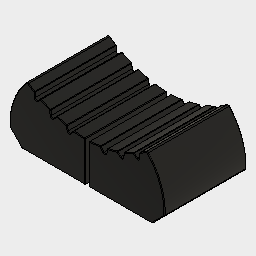
ALPS Fader Knob (Autodesk Fusion 360 design; units mm, degrees)
Autodesk Fusion 360 part; units mm, degrees
sketch "Skizze1" plane through (0, 0, 0) normal (0, 1, 0) x (1, 0, 0)
  line L0 (0, 0) -> (10.3, 0)
  line L1 (10.3, 0) -> (12.3, -2)
  line L2 (0, -11.0044) -> (0, 4.9956) construction
  arc A0 (9.5, -9.5) -> (12.3, -2) centre (1.806, -2.3549) ccw
  arc A1 (9.5, -9.5) -> (0, -6.3) centre (-0.6023, -23.7896) ccw
  line L3 (-0.9062, -6.3) -> (0.9938, -6.3) construction
  arc A2 (-12.3, -2) -> (-9.5, -9.5) centre (-1.806, -2.3549) ccw
  arc A3 (0, -6.3) -> (-9.5, -9.5) centre (0.6023, -23.7896) ccw
  line L4 (0, 0) -> (-10.3, 0)
  line L5 (-10.3, 0) -> (-12.3, -2)
  dimension "d1" = 135
  dimension "d2" = 6.3
  dimension "d3" = 2
  dimension "d4" = 10.3
  dimension "d5" = 10.5
  dimension "d6" = 17.5
  dimension "d7" = 9.5
  dimension "d8" = 9.5
  measures "d1" angle of L0 L1
  measures "d2" distance of L0.start L3
  measures "d3" distance of L0 L1.end
  measures "d4" distance of L0.start L0.end
  measures "d5" radius of A0
  measures "d6" radius of A1
  measures "d7" distance of L2 A0.start
  measures "d8" distance of L0 A0.start
extrude "Extrusion1" add sketch "Skizze1" along normal mid plane 13
sketch "Skizze2" plane through (0, -6.5, 0) normal (0, -1, 0) x (1, 0, 0)
  line L0 (-10.3, 0) -> (10.3, 0)
  line L1 (10.3, 0) -> (12.3, 2)
  arc A0 (12.3, 2) -> (9.5, 9.5) centre (1.806, 2.3549) ccw
  arc A1 (0, 6.3) -> (9.5, 9.5) centre (-0.6023, 23.7896) ccw
  arc A2 (-9.5, 9.5) -> (0, 6.3) centre (0.6023, 23.7896) ccw
  arc A3 (-9.5, 9.5) -> (-12.3, 2) centre (-1.806, 2.3549) ccw
  line L2 (-12.3, 2) -> (-10.3, 0)
  arc A4 (-9.5, 9.5) -> (0, 6.3) centre (0.6023, 23.7896) ccw
  arc A5 (0, 6.3) -> (9.5, 9.5) centre (-0.6023, 23.7896) ccw
  line L3 (10.3, 0) -> (-10.3, 0)
  line L4 (-10.3, 0) -> (-12.3, 2)
  arc A6 (-9.5, 9.5) -> (-12.3, 2) centre (-1.806, 2.3549) ccw
  arc A7 (-9.5, 9.5) -> (0, 6.3) centre (0.6023, 23.7896) ccw
  arc A8 (0, 6.3) -> (9.5, 9.5) centre (-0.6023, 23.7896) ccw
  arc A9 (12.3, 2) -> (9.5, 9.5) centre (1.806, 2.3549) ccw
  line L5 (12.3, 2) -> (10.3, 0)
  line L6 (-8.3055, 8.7264) -> (-8.2923, 7.9551)
  line L7 (-7.8783, 7.7707) -> (-7.3709, 8.2115)
  arc A10 (-8.2923, 7.9551) -> (-7.8783, 7.7707) centre (-8.0423, 7.9594) ccw
  line L8 (-5.8203, 7.5108) -> (-5.7421, 6.772)
  arc A11 (-5.7421, 6.772) -> (-5.3135, 6.6248) centre (-5.4935, 6.7983) ccw
  line L9 (-5.3135, 6.6248) -> (-4.8095, 7.1475)
  line L10 (-2.6202, 5.8954) -> (-2.1282, 6.504)
  arc A12 (-3.06, 6.0046) -> (-2.6202, 5.8954) centre (-2.8147, 6.0525) ccw
  line L11 (-3.1972, 6.7071) -> (-3.06, 6.0046)
  line L12 (-0.35, 6.3156) -> (-0.35, 5.5)
  line L13 (-0.35, 5.5) -> (0.35, 5.5)
  line L14 (0.35, 5.5) -> (0.35, 6.3156)
  line L15 (1.75, 0) -> (22.5, 0)
  line L16 (0, 1.75) -> (0, 22.5)
  line L17 (7.8783, 7.7707) -> (7.3709, 8.2115)
  arc A13 (7.8783, 7.7707) -> (8.2923, 7.9551) centre (8.0423, 7.9594) ccw
  line L18 (8.3055, 8.7264) -> (8.2923, 7.9551)
  line L19 (5.3135, 6.6248) -> (4.8095, 7.1475)
  arc A14 (5.3135, 6.6248) -> (5.7421, 6.772) centre (5.4935, 6.7983) ccw
  line L20 (5.8203, 7.5108) -> (5.7421, 6.772)
  line L21 (2.6202, 5.8954) -> (2.1282, 6.504)
  arc A15 (2.6202, 5.8954) -> (3.06, 6.0046) centre (2.8147, 6.0525) ccw
  line L22 (3.1972, 6.7071) -> (3.06, 6.0046)
  dimension "d12" = 50
  dimension "d13" = 0.25
  dimension "d14" = 50
  dimension "d15" = 0.25
  dimension "d16" = 50
  dimension "d17" = 0.25
  dimension "d18" = 0.8
  dimension "d29" = 0.7
  measures "d12" angle of L6 L7
  measures "d13" radius of A10
  measures "d14" angle of L8 L9
  measures "d15" radius of A11
  measures "d16" angle of L10 L11
  measures "d17" radius of A12
  measures "d18" distance of A1.start L13
  measures "d29" distance of L12 L14
extrude "Extrusion2" cut sketch "Skizze2" against normal blind 13 contours A2 A4 A7 L6 L7 A10 | A1 A5 A8 L17 A13 L18 | A2 A4 A7 L8 A11 L9 | A1 A5 A8 L19 A14 L20 | A2 A4 A7 L10 A12 L11 | A1 A5 A8 L21 A15 L22 | A2 A4 A7 L12 L13 L16 | A1 A5 A8 L13 L14 L16
fillet "Abrundung1" radius 0.1 14 edges at (-8.3055, 0, 8.7264) (-7.3709, 0, 8.2115) (-5.8203, 0, 7.5108) (-4.8095, 0, 7.1475) (-3.1972, 0, 6.7071) (-2.1282, 0, 6.504) (-0.35, 0, 6.3156) (0.35, 0, 6.3156) (2.1282, 0, 6.504) (3.1972, 0, 6.7071) (4.8095, 0, 7.1475) (5.8203, 0, 7.5108) (7.3709, 0, 8.2115) (8.3055, 0, 8.7264)
fillet "Abrundung2" radius 0.25 6 edges at (-9.5, 0, 9.5) (9.5, 0, 9.5) (12.3, 0, 2) (10.3, 0, 0) (-12.3, 0, 2) (-10.3, 0, 0)
sketch "Skizze4" plane through (0, 0, 0) normal (0, 0, 1) x (1, 0, 0)
  line L0 (1.75, 0) -> (22.5, 0)
  line L1 (-0.35, -6.5) -> (0.35, -6.5)
  line L2 (0.35, -6.5) -> (0.35, -5.8)
  line L3 (0.35, -5.8) -> (-0.35, -5.8)
  line L4 (-0.35, -5.8) -> (-0.35, -6.5)
  line L5 (0.35, -6.5) -> (-0.35, -6.5)
  line L6 (-10.1964, -6.5) -> (10.1964, -6.5)
  line L7 (0, 1.75) -> (0, 22.5)
  line L8 (0.35, 6.5) -> (0.35, 5.8)
  line L9 (-0.35, 5.8) -> (-0.35, 6.5)
  line L10 (-0.35, 6.5) -> (0.35, 6.5)
  line L11 (0.35, 6.5) -> (-0.35, 6.5)
  line L12 (-10.1964, 6.5) -> (10.1964, 6.5)
  line L13 (0.35, 5.8) -> (-0.35, 5.8)
  dimension "d25" = 0.7
  dimension "d26" = 0.7
  measures "d25" distance of L1 L3
  measures "d26" distance of L2 L4
extrude "Extrusion3" cut sketch "Skizze4" along normal blind 6
sketch "Skizze5" plane through (0, 0, 0) normal (0, 0, 1) x (1, 0, 0)
  line L0 (1.75, 0) -> (22.5, 0)
  line L1 (0, 1.75) -> (0, 22.5)
  line L2 (-2, -0.6) -> (2, -0.6)
  line L3 (2, -0.6) -> (2, 0.6)
  line L4 (2, 0.6) -> (-2, 0.6)
  line L5 (-2, 0.6) -> (-2, -0.6)
  dimension "d30" = 4
  dimension "d31" = 1.2
  measures "d30" distance of L3 L5
  measures "d31" distance of L2 L4
extrude "Extrusion4" cut sketch "Skizze5" along normal blind 5
sketch "Skizze6" plane through (0, 0, 0) normal (0, 0, 1) x (1, 0, 0)
  line L0 (-8.75, -4) -> (8.75, -4)
  line L1 (8.75, -4) -> (8.75, -1.5)
  line L2 (8.75, -1.5) -> (-8.75, -1.5)
  line L3 (-8.75, -1.5) -> (-8.75, -4)
  line L4 (1.75, 0) -> (22.5, 0)
  line L5 (0, 1.75) -> (0, 22.5)
  line L6 (-8.75, 1.5) -> (8.75, 1.5)
  line L7 (8.75, 1.5) -> (8.75, 4)
  line L8 (8.75, 4) -> (-8.75, 4)
  line L9 (-8.75, 4) -> (-8.75, 1.5)
  line L10 (-8.75, -1) -> (-2.9, -1)
  line L11 (-2.9, -1) -> (-2.9, 1)
  line L12 (-2.9, 1) -> (-8.75, 1)
  line L13 (-8.75, 1) -> (-8.75, -1)
  line L14 (2.9, 1) -> (8.75, 1)
  line L15 (8.75, -1) -> (2.9, -1)
  line L16 (2.9, -1) -> (2.9, 1)
  line L17 (8.75, 1) -> (8.75, -1)
  dimension "d34" = 17.5
  dimension "d35" = 2.5
  dimension "d36" = 1.5
  dimension "d37" = 2.5
  dimension "d38" = 17.5
  dimension "d39" = 1.5
  dimension "d40" = 2.9
  dimension "d42" = 2
  measures "d34" distance of L0.start L0.end
  measures "d35" distance of L0 L2
  measures "d36" distance of L2 L4
  measures "d37" distance of L6 L8
  measures "d38" distance of L7 L9
  measures "d39" distance of L4 L6
  measures "d40" distance of L5 L11
  measures "d42" distance of L10 L12
extrude "Extrusion5" cut sketch "Skizze6" along normal blind 5
fillet "Abrundung3" radius 0.1 108 edges at (-0.35, -6.5, 3.1106) (-0.3772, -6.5, 6.2897) (-1.2598, -6.5, 6.389) (-2.1228, -6.5, 6.4895) (-2.3924, -6.5, 6.1772) (-2.8749, -6.5, 5.8099) (-3.1223, -6.5, 6.3238) (-3.211, -6.5, 6.6934) (-4.01, -6.5, 6.9084) (-4.8053, -6.5, 7.1301) (-5.0832, -6.5, 6.8637) (-5.5747, -6.5, 6.5619) (-5.778, -6.5, 7.1113) (-5.8337, -6.5, 7.5005) (-6.601, -6.5, 7.8409) (-7.3685, -6.5, 8.191) (-7.6501, -6.5, 7.969) (-8.1441, -6.5, 7.731) (-8.2984, -6.5, 8.3128) (-8.318, -6.5, 8.719) (-8.8423, -6.5, 9.057) (-9.4928, -6.5, 9.4174) (-11.664, -6.5, 5.9702) (-12.2828, -6.5, 2.0081) (-11.3015, -6.5, 1.0015) (-10.2921, -6.5, 0.019) (-5.2732, -6.5, 0) (5.2732, -6.5, 0) (10.2921, -6.5, 0.019) (11.3015, -6.5, 1.0015) (12.2828, -6.5, 2.0081) (11.664, -6.5, 5.9702) (9.4928, -6.5, 9.4174) (8.8423, -6.5, 9.057) (8.318, -6.5, 8.719) (8.2984, -6.5, 8.3128) (8.1441, -6.5, 7.731) (7.6501, -6.5, 7.969) (7.3685, -6.5, 8.191) (6.601, -6.5, 7.8409) (5.8337, -6.5, 7.5005) (5.778, -6.5, 7.1113) (5.5747, -6.5, 6.5619) (5.0832, -6.5, 6.8637) (4.8053, -6.5, 7.1301) (4.01, -6.5, 6.9084) (3.211, -6.5, 6.6934) (3.1223, -6.5, 6.3238) (2.8749, -6.5, 5.8099) (2.3924, -6.5, 6.1772) (2.1228, -6.5, 6.4895) (1.2598, -6.5, 6.389) (0.3772, -6.5, 6.2897) (0.35, -6.5, 3.1106) (-5.2732, 6.5, 0) (-10.2921, 6.5, 0.019) (-11.3015, 6.5, 1.0015) (-12.2828, 6.5, 2.0081) (-11.664, 6.5, 5.9702) (-9.4928, 6.5, 9.4174) (-8.8423, 6.5, 9.057) (-8.318, 6.5, 8.719) (-8.2984, 6.5, 8.3128) (-8.1441, 6.5, 7.731) (-7.6501, 6.5, 7.969) (-7.3685, 6.5, 8.191) (-6.601, 6.5, 7.8409) (-5.8337, 6.5, 7.5005) (-5.778, 6.5, 7.1113) (-5.5747, 6.5, 6.5619) (-5.0832, 6.5, 6.8637) (-4.8053, 6.5, 7.1301) (-4.01, 6.5, 6.9084) (-3.211, 6.5, 6.6934) (-3.1223, 6.5, 6.3238) (-2.8749, 6.5, 5.8099) (-2.3924, 6.5, 6.1772) (-2.1228, 6.5, 6.4895) (-1.2598, 6.5, 6.389) (-0.3772, 6.5, 6.2897) (-0.35, 6.5, 3.1106) (0.35, 6.5, 3.1106) (0.3772, 6.5, 6.2897) (1.2598, 6.5, 6.389) (2.1228, 6.5, 6.4895) (2.3924, 6.5, 6.1772) (2.8749, 6.5, 5.8099) (3.1223, 6.5, 6.3238) (3.211, 6.5, 6.6934) (4.01, 6.5, 6.9084) (4.8053, 6.5, 7.1301) (5.0832, 6.5, 6.8637) (5.5747, 6.5, 6.5619) (5.778, 6.5, 7.1113) (5.8337, 6.5, 7.5005) (6.601, 6.5, 7.8409) (7.3685, 6.5, 8.191) (7.6501, 6.5, 7.969) (8.1441, 6.5, 7.731) (8.2984, 6.5, 8.3128) (8.318, 6.5, 8.719) (8.8423, 6.5, 9.057) (9.4928, 6.5, 9.4174) (11.664, 6.5, 5.9702) (12.2828, 6.5, 2.0081) (11.3015, 6.5, 1.0015) (10.2921, 6.5, 0.019) (5.2732, 6.5, 0)
sketch "Skizze7" plane through (0, 0, 0) normal (0, 0, -1) x (1, 0, 0)
  line L0 (-2.9, -1) -> (-8.75, -1)
  line L1 (-8.75, -1) -> (-8.75, 1)
  line L2 (-8.75, 1) -> (-2.9, 1)
  line L3 (-2.9, 1) -> (-2.9, -1)
  line L4 (8.75, 1.5) -> (-8.75, 1.5)
  line L5 (-8.75, 1.5) -> (-8.75, 4)
  line L6 (-8.75, 4) -> (8.75, 4)
  line L7 (8.75, 4) -> (8.75, 1.5)
  line L8 (8.75, -4) -> (-8.75, -4)
  line L9 (-8.75, -4) -> (-8.75, -1.5)
  line L10 (-8.75, -1.5) -> (8.75, -1.5)
  line L11 (8.75, -1.5) -> (8.75, -4)
  line L12 (8.75, 1) -> (8.75, -1)
  line L13 (8.75, -1) -> (2.9, -1)
  line L14 (2.9, -1) -> (2.9, 1)
  line L15 (2.9, 1) -> (8.75, 1)
  line L16 (2, -0.6) -> (-2, -0.6)
  line L17 (-2, -0.6) -> (-2, 0.6)
  line L18 (-2, 0.6) -> (2, 0.6)
  line L19 (2, 0.6) -> (2, -0.6)
  line L20 (0.35, -6.4) -> (10.1964, -6.4)
  line L21 (10.1964, -6.4) -> (10.1964, 6.4)
  line L22 (10.1964, 6.4) -> (0.35, 6.4)
  line L23 (0.35, 6.4) -> (0.35, 5.8)
  line L24 (0.35, 5.8) -> (-0.35, 5.8)
  line L25 (-0.35, 5.8) -> (-0.35, 6.4)
  line L26 (-0.35, 6.4) -> (-10.1964, 6.4)
  line L27 (-10.1964, 6.4) -> (-10.1964, -6.4)
  line L28 (-10.1964, -6.4) -> (-0.35, -6.4)
  line L29 (-0.35, -6.4) -> (-0.35, -5.8)
  line L30 (-0.35, -5.8) -> (0.35, -5.8)
  line L31 (0.35, -5.8) -> (0.35, -6.4)
  line L32 (-9.6964, -5.9) -> (-0.85, -5.9)
  line L33 (-0.85, -5.9) -> (-0.85, -5.3)
  line L34 (-0.85, -5.3) -> (0.85, -5.3)
  line L35 (0.85, -5.3) -> (0.85, -5.9)
  line L36 (0.85, -5.9) -> (9.6964, -5.9)
  line L37 (9.6964, -5.9) -> (9.6964, 5.9)
  line L38 (9.6964, 5.9) -> (0.85, 5.9)
  line L39 (0.85, 5.9) -> (0.85, 5.3)
  line L40 (0.85, 5.3) -> (-0.85, 5.3)
  line L41 (-0.85, 5.3) -> (-0.85, 5.9)
  line L42 (-0.85, 5.9) -> (-9.6964, 5.9)
  line L43 (-9.6964, 5.9) -> (-9.6964, -5.9)
  dimension "d47" = 0.5
extrude "Extrusion6" cut sketch "Skizze7" against normal blind 0.1 contours L32 L33 L34 L35 L36 L37 L38 L39 L40 L41 L42 L43
